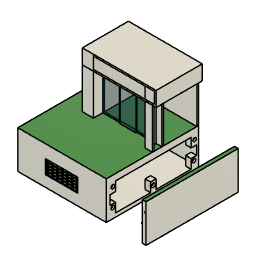
Test_Coffret_Conception Maison Energetique_1 v6(2) (Autodesk Fusion 360 design; units mm, degrees)
Autodesk Fusion 360 part; units mm, degrees
note: some values were not read from the file. Chosen so that the rebuilt part matches the saved one: which bodies a step acts on. Set by a fixed rule: which sketch regions a step uses.
(part 1 of 3)
sketch "Esquisse1" plane through (0, 0, 0) normal (0, 1, 0) x (1, 0, 0)
  line L0 (0, 0) -> (500, 0)
  line L1 (500, 0) -> (500, 500)
  line L2 (500, 500) -> (0, 500)
  line L3 (0, 500) -> (0, 0)
  dimension "d1" = 500
  dimension "d2" = 500
  constraint horizontal L0
  constraint vertical L1
  constraint horizontal L2
  constraint vertical L3
  constraint coincident L0.start L3.end
  measures "d1" distance of L0.start L0.end
  measures "d2" distance of L0.start L2.end
extrude "Extrusion1" add sketch "Esquisse1" along normal blind 40 makes body 1
sketch "Esquisse2" plane through (0, 40, 0) normal (0, 1, 0) x (-1, 0, 0)
  line L0 (0, -500) -> (0, 0)
  line L1 (0, 0) -> (-500, 0)
  line L2 (-500, 0) -> (-500, -500)
  line L3 (-500, -500) -> (0, -500)
  line L4 (-75, -500) -> (-500, -500)
  line L5 (-500, -500) -> (-500, -250)
  line L6 (-500, -250) -> (-75, -250)
  line L7 (-75, -250) -> (-75, -500)
  line L8 (-480, -480) -> (-480, -270)
  line L9 (-480, -270) -> (-95, -270)
  line L10 (-95, -270) -> (-95, -480)
  line L11 (-95, -480) -> (-480, -480)
  dimension "d5" = 20
  constraint horizontal L4
  constraint vertical L5
  constraint horizontal L6
  constraint vertical L7
  constraint midpoint L2 L5.end
  constraint coincident L3 L4.start
extrude "Extrusion2" add sketch "Esquisse2" along normal blind 400 contours L2 L3 L4 L5 L6 L7 bodies 1
sketch "Esquisse3" plane through (0, 440, 0) normal (0, 1, 0) x (-1, 0, 0)
  line L0 (-95, -270) -> (-95, -480)
  line L1 (-95, -480) -> (-480, -480)
  line L2 (-480, -480) -> (-480, -270)
  line L3 (-480, -270) -> (-95, -270)
  line L4 (-75, -250) -> (-500, -250)
  line L5 (-500, -250) -> (-500, -500)
  line L6 (-500, -500) -> (-75, -500)
  line L7 (-75, -500) -> (-75, -250)
  line L8 (-75, -500) -> (-500, -500)
  line L9 (-500, -500) -> (-500, -200)
  line L10 (-500, -200) -> (-75, -200)
  line L11 (-75, -200) -> (-75, -500)
  constraint horizontal L8
  constraint vertical L9
  constraint horizontal L10
  constraint vertical L11
  constraint coincident L6.end L7.start
extrude "Extrusion3" add sketch "Esquisse3" against normal blind 20 separate body contours L0 L1 L2 L3 | L4 L5 L6 L7 L8 L9 L11 | L4 L9 L10 L11 makes body 2
copy_body "Copier/Coller des corps1" bodies 2 makes body 3
move_body "Déplacer1" bodies 3 to x (1, 0, 0) y (0, 1, 0) z (0, 0, 1) at (0, -100, 0)
sketch "Esquisse4" plane through (0, 0, -250) normal (0, 0, 1) x (1, 0, 0)
  line L0 (75, 40) -> (500, 40)
  line L1 (500, 40) -> (500, 440)
  line L2 (500, 440) -> (75, 440)
  line L3 (75, 440) -> (75, 40)
  line L4 (75, 420) -> (500, 420)
  line L5 (500, 420) -> (500, 340)
  line L6 (500, 340) -> (75, 340)
  line L7 (75, 340) -> (75, 420)
  constraint horizontal L4
  constraint vertical L5
  constraint horizontal L6
  constraint vertical L7
  constraint coincident L1 L5.end
  constraint coincident L3 L4.start
extrude "Extrusion4" add sketch "Esquisse4" along normal blind 50 contours L1 L3 L4 L5 L6 L7 bodies 1 2 3
sketch "Esquisse5" plane through (0, 0, -200) normal (0, 0, 1) x (1, 0, 0)
  line L0 (500, 440) -> (75, 440)
  line L1 (75, 440) -> (75, 420)
  line L2 (75, 420) -> (75, 320)
  line L3 (75, 320) -> (500, 320)
  line L4 (500, 320) -> (500, 420)
  line L5 (500, 420) -> (500, 440)
  line L6 (95, 420) -> (95, 340)
  line L7 (95, 340) -> (480, 340)
  line L8 (480, 340) -> (480, 420)
  line L9 (480, 420) -> (95, 420)
  dimension "d12" = -20
extrude "Extrusion5" cut sketch "Esquisse5" against normal blind 280 contours L6 L7 L8 L9 bodies 1
ref_plane "Plan de construction1" through (287.5, 320, -225) normal (0, -1, 0) x (0, 0, -1)
split "Scinder1" by plane through (287.5, 320, -225) normal (0, -1, 0) bodies 1 makes body 4 at (166.6667, 0, -333.3333)
sketch "Esquisse6" plane through (0, 0, -200) normal (0, 0, 1) x (1, 0, 0)
  line L0 (95, 340) -> (95, 420)
  line L1 (95, 420) -> (480, 420)
  line L2 (480, 420) -> (480, 340)
  line L3 (480, 340) -> (95, 340)
  line L4 (500, 440) -> (75, 440)
  line L5 (75, 440) -> (75, 420)
  line L6 (75, 420) -> (75, 320)
  line L7 (75, 320) -> (500, 320)
  line L8 (500, 320) -> (500, 420)
  line L9 (500, 420) -> (500, 440)
  line L10 (95, 420) -> (480, 420)
  line L11 (480, 420) -> (480, 340)
  line L12 (480, 340) -> (95, 340)
  line L13 (95, 340) -> (95, 420)
  constraint horizontal L10
  constraint vertical L11
  constraint horizontal L12
  constraint vertical L13
  constraint coincident L2.end L3.start
  constraint coincident L0.end L1.start
extrude "Extrusion6" add sketch "Esquisse6" against normal blind 20 separate body contours L0 L1 L2 L3 L10 L11 L12 L13 makes body 5
ref_plane "Plan de construction2" through (250, 40, -250) normal (0, 1, 0) x (0, 0, 1)
split "Scinder2" by plane through (250, 40, -250) normal (0, 1, 0) bodies 4 makes body 6 at (358.3333, 133.3333, -500)
sketch "Esquisse7" plane through (0, 0, -250) normal (0, 0, 1) x (1, 0, 0)
  line L0 (500, 320) -> (75, 320)
  line L1 (75, 320) -> (75, 40)
  line L2 (75, 40) -> (500, 40)
  line L3 (500, 40) -> (500, 320)
  line L4 (188.1968, 40) -> (363.1968, 40)
  line L5 (363.1968, 40) -> (363.1968, 250)
  line L6 (363.1968, 250) -> (188.1968, 250)
  line L7 (188.1968, 250) -> (188.1968, 40)
  dimension "d19" = 175
  dimension "d20" = 210
  constraint horizontal L4
  constraint vertical L5
  constraint horizontal L6
  constraint vertical L7
  constraint coincident L2 L4.start
  measures "d19" distance of L4.start L4.end
  measures "d20" distance of L4.start L6.end
extrude "Extrusion7" cut sketch "Esquisse7" against normal blind 15 contours L2 L4 L5 L6 L7 bodies 6
sketch "Esquisse8" plane through (0, 0, -265) normal (0, 0, 1) x (1, 0, 0)
  line L0 (188.1968, 250) -> (188.1968, 40)
  line L1 (188.1968, 40) -> (363.1968, 40)
  line L2 (363.1968, 40) -> (363.1968, 250)
  line L3 (363.1968, 250) -> (188.1968, 250)
extrude "Extrusion8" add sketch "Esquisse8" along normal blind 20 bodies 6
sketch "Esquisse9" plane through (0, 40, 0) normal (0, 1, 0) x (-1, 0, 0)
  line L0 (-500, -500) -> (0, -500)
  line L1 (0, -500) -> (0, 0)
  line L2 (0, 0) -> (-500, 0)
  line L3 (-500, 0) -> (-500, -500)
  line L4 (-480, -270) -> (-450, -270)
  line L5 (-450, -270) -> (-450, -300)
  line L6 (-450, -300) -> (-480, -300)
  line L7 (-480, -300) -> (-480, -270)
  line L8 (-500, -320) -> (-500, -250)
  line L9 (-500, -250) -> (-430, -250)
  line L10 (-430, -250) -> (-430, -320)
  line L11 (-430, -320) -> (-500, -320)
  dimension "d25" = 30
  dimension "d26" = 30
  dimension "d27" = -20
  constraint horizontal L4
  constraint vertical L5
  constraint horizontal L6
  constraint vertical L7
  measures "d25" distance of L4.start L4.end
  measures "d26" distance of L4.start L6.end
extrude "Extrusion9" add sketch "Esquisse9" along normal blind 280 separate body contours L3 L8 L9 L10 L11 makes body 7
sketch "Esquisse10" plane through (0, 0, 0) normal (0, -1, 0) x (1, 0, 0)
  line L0 (0, 0) -> (0, -500)
  line L1 (0, -500) -> (500, -500)
  line L2 (500, -500) -> (500, 0)
  line L3 (500, 0) -> (0, 0)
  line L4 (480, -480) -> (480, -20)
  line L5 (480, -20) -> (20, -20)
  line L6 (20, -20) -> (20, -480)
  line L7 (20, -480) -> (480, -480)
  dimension "d30" = -20
extrude "Extrusion10" add sketch "Esquisse10" along normal blind 100 separate body makes body 8
sketch "Esquisse11" plane through (0, -100, 0) normal (0, -1, 0) x (1, 0, 0)
  line L0 (480, -480) -> (20, -480)
  line L1 (20, -480) -> (20, -20)
  line L2 (20, -20) -> (480, -20)
  line L3 (480, -20) -> (480, -480)
  line L4 (500, 0) -> (0, 0)
  line L5 (0, 0) -> (0, -500)
  line L6 (0, -500) -> (500, -500)
  line L7 (500, -500) -> (500, 0)
  line L8 (0, 0) -> (500, 0)
  line L9 (500, 0) -> (500, -500)
  line L10 (500, -500) -> (0, -500)
  line L11 (0, -500) -> (0, 0)
  constraint horizontal L8
  constraint vertical L9
  constraint horizontal L10
  constraint vertical L11
  constraint coincident L6.end L7.start
  constraint coincident L4.end L5.start
extrude "Extrusion11" add sketch "Esquisse11" along normal blind 20 separate body contours L0 L1 L2 L3 | L4 L5 L6 L7 L8 L9 L10 L11 makes body 9
sketch "Esquisse12" plane through (0, 0, 0) normal (0, -1, 0) x (1, 0, 0)
  line L0 (0, 0) -> (0, -500)
  line L1 (0, -500) -> (500, -500)
  line L2 (500, -500) -> (500, 0)
  line L3 (500, 0) -> (0, 0)
  line L4 (20, -171) -> (480.0003, -171)
  line L5 (480.0003, -171) -> (480.0003, -151)
  line L6 (480.0003, -151) -> (20, -151)
  line L7 (20, -151) -> (20, -171)
  dimension "d35" = 20
  constraint horizontal L4
  constraint vertical L5
  constraint horizontal L6
  constraint vertical L7
  measures "d35" distance of L4.start L6.end
extrude "Extrusion12" add sketch "Esquisse12" along normal blind 100 separate body contours L4 L5 L6 L7 makes body 10
move_body "Déplacer2" bodies 10 to x (1, 0, 0) y (0, 1, 0) z (0, 0, 1) at (0, 0, -50)
sketch "Esquisse13" plane through (0, 0, 0) normal (0, 0, 1) x (1, 0, 0)
  line L0 (500, 0) -> (0, 0)
  line L1 (0, 0) -> (0, -100)
  line L2 (0, -100) -> (500, -100)
  line L3 (500, -100) -> (500, 0)
  line L4 (480, -80) -> (480, -20)
  line L5 (480, -20) -> (20, -20)
  line L6 (20, -20) -> (20, -80)
  line L7 (20, -80) -> (480, -80)
  dimension "d38" = -20
extrude "Extrusion13" cut sketch "Esquisse13" against normal blind 20 contours L4 L5 L6 L7 bodies 8
sketch "Esquisse14" plane through (0, 0, -201) normal (0, 0, 1) x (1, 0, 0)
  line L0 (480.0003, 0) -> (20, 0)
  line L1 (20, 0) -> (20, -100)
  line L2 (20, -100) -> (480.0003, -100)
  line L3 (480.0003, -100) -> (480.0003, 0)
  line L4 (0, -50) -> (500, -50)
  line L5 (250, -50) -> (200, -50)
  line L6 (250, -50) -> (300, -50)
  line L7 (200, -50) -> (200, -25)
  line L8 (200, -50) -> (200, -75)
  line L9 (200, -25) -> (300, -25)
  line L10 (300, -25) -> (300, -75)
  line L11 (300, -75) -> (200, -75)
  line L12 (200, -75) -> (200, -25)
  dimension "d41" = 50
  dimension "d42" = 50
  dimension "d43" = 25
  dimension "d45" = 25
  constraint perpendicular L3 L4
  constraint midpoint L4 L5.start
  constraint parallel L4 L5
  constraint parallel L4 L6
  constraint perpendicular L0 L7
  constraint perpendicular L4 L8
  constraint horizontal L9
  constraint vertical L10
  constraint horizontal L11
  constraint vertical L12
  measures "d41" distance of L5.start L5.end
  measures "d42" distance of L5.start L6.end
  measures "d43" distance of L5.end L7.end
  measures "d45" distance of L5.end L8.end
extrude "Extrusion14" cut sketch "Esquisse14" against normal blind 20 contours L4 L5 L6 L8 L10 L11 L12 | L4 L5 L6 L7 L9 L10 L12 bodies 10
sketch "Esquisse15" plane through (0, 0, -480) normal (0, 0, 1) x (1, 0, 0)
  line L0 (480, 0) -> (20, 0)
  line L1 (20, 0) -> (20, -100)
  line L2 (20, -100) -> (480, -100)
  line L3 (480, -100) -> (480, 0)
  line L4 (230, -30) -> (270, -30)
  line L5 (270, -30) -> (270, -70)
  line L6 (270, -70) -> (230, -70)
  line L7 (230, -70) -> (230, -30)
  spline S0 degree 5 poles (250, -50) (249.4889, -49.5996) (248.5057, -48.7988) (247.1484, -47.5977) (245.5774, -45.9965) (244.0392, -43.9954) (242.9669, -41.9947) (242.4027, -39.9944) (242.3763, -37.9947) (242.8764, -35.9953) (243.8673, -33.9965) (245.0225, -32.3977) (246.0802, -31.1988) (246.8689, -30.3996) (247.2842, -30) knots 0 0 0 0 0 0 0.1 0.2 0.3 0.4 0.5 0.6 0.7 0.8 0.9 1 1 1 1 1 1
  spline S1 degree 5 poles (247.2842, -30) (247.159, -30.2933) (246.9356, -30.9388) (246.6822, -32.0838) (246.5187, -33.9882) (246.7472, -37.3065) (247.4945, -41.1841) (248.532, -45.1258) (249.4696, -48.2864) (250, -50) knots 0 0 0 0 0 0 0.2 0.4 0.6 0.8 1 1 1 1 1 1
  line L8 (248.6567, -45.6598) -> (251.3433, -54.3402)
  spline S2 degree 5 poles (249.6809, -50.207) (249.7158, -49.5586) (249.8078, -48.294) (250.0132, -46.4932) (250.4237, -44.2879) (251.1806, -41.88) (252.2045, -39.8541) (253.5194, -38.2446) (255.1423, -37.076) (257.0669, -36.3389) (259.2727, -36.0041) (261.2449, -36.0334) (262.8337, -36.2121) (263.9407, -36.3998) (264.5063, -36.5108) knots 0 0 0 0 0 0 0.1 0.2 0.3 0.4 0.5 0.6 0.7 0.8 0.9 1 1 1 1 1 1
  spline S3 degree 5 poles (264.5063, -36.5108) (264.1941, -36.5764) (263.5373, -36.7637) (262.454, -37.2128) (260.8003, -38.1712) (258.2131, -40.2617) (255.4654, -43.098) (252.8317, -46.2087) (250.7805, -48.7896) (249.6809, -50.207) knots 0 0 0 0 0 0 0.2 0.4 0.6 0.8 1 1 1 1 1 1
  line L9 (252.4658, -46.6172) -> (246.8961, -53.7967)
  spline S4 degree 5 poles (250, -50) (249.4889, -49.5996) (248.5057, -48.7988) (247.1484, -47.5977) (245.5774, -45.9965) (244.0392, -43.9954) (242.9669, -41.9947) (242.4027, -39.9944) (242.3763, -37.9947) (242.8764, -35.9953) (243.8673, -33.9965) (245.0225, -32.3977) (246.0802, -31.1988) (246.8689, -30.3996) (247.2842, -30) knots 0 0 0 0 0 0 0.1 0.2 0.3 0.4 0.5 0.6 0.7 0.8 0.9 1 1 1 1 1 1
  spline S5 degree 5 poles (247.2842, -30) (247.159, -30.2933) (246.9356, -30.9388) (246.6822, -32.0838) (246.5187, -33.9882) (246.7472, -37.3065) (247.4945, -41.1841) (248.532, -45.1258) (249.4696, -48.2864) (250, -50) knots 0 0 0 0 0 0 0.2 0.4 0.6 0.8 1 1 1 1 1 1
  line L10 (248.6567, -45.6598) -> (251.3433, -54.3402)
  spline S6 degree 5 poles (264.5063, -36.5108) (264.1941, -36.5764) (263.5373, -36.7637) (262.454, -37.2128) (260.8003, -38.1712) (258.2131, -40.2617) (255.4654, -43.098) (252.8317, -46.2087) (250.7805, -48.7896) (249.6809, -50.207) knots 0 0 0 0 0 0 0.2 0.4 0.6 0.8 1 1 1 1 1 1
  line L11 (252.4658, -46.6172) -> (246.8961, -53.7967)
  spline S7 degree 5 poles (249.6809, -50.207) (249.7158, -49.5586) (249.8078, -48.294) (250.0132, -46.4932) (250.4237, -44.2879) (251.1806, -41.88) (252.2045, -39.8541) (253.5194, -38.2446) (255.1423, -37.076) (257.0669, -36.3389) (259.2727, -36.0041) (261.2449, -36.0334) (262.8337, -36.2121) (263.9407, -36.3998) (264.5063, -36.5108) knots 0 0 0 0 0 0 0.1 0.2 0.3 0.4 0.5 0.6 0.7 0.8 0.9 1 1 1 1 1 1
  spline S8 degree 5 poles (250.0313, -49.9578) (250.4317, -49.4466) (251.2325, -48.4635) (252.4336, -47.1062) (254.0348, -45.5352) (256.0359, -43.9969) (258.0366, -42.9247) (260.0369, -42.3604) (262.0367, -42.334) (264.036, -42.8342) (266.0349, -43.8251) (267.6336, -44.9803) (268.8326, -46.038) (269.6318, -46.8267) (270.0313, -47.242) knots 0 0 0 0 0 0 0.1 0.2 0.3 0.4 0.5 0.6 0.7 0.8 0.9 1 1 1 1 1 1
  spline S9 degree 5 poles (270.0313, -47.242) (269.738, -47.1167) (269.0925, -46.8934) (267.9476, -46.64) (266.0432, -46.4765) (262.7249, -46.705) (258.8472, -47.4523) (254.9056, -48.4898) (251.745, -49.4274) (250.0313, -49.9578) knots 0 0 0 0 0 0 0.2 0.4 0.6 0.8 1 1 1 1 1 1
  line L12 (254.3715, -48.6145) -> (245.6911, -51.301)
  spline S10 degree 5 poles (263.5206, -64.464) (263.4549, -64.1519) (263.2676, -63.4951) (262.8185, -62.4118) (261.8601, -60.758) (259.7696, -58.1709) (256.9334, -55.4232) (253.8226, -52.7894) (251.2417, -50.7382) (249.8244, -49.6387) knots 0 0 0 0 0 0 0.2 0.4 0.6 0.8 1 1 1 1 1 1
  line L13 (253.4142, -52.4235) -> (246.2346, -46.8539)
  spline S11 degree 5 poles (249.8244, -49.6387) (250.4727, -49.6735) (251.7374, -49.7656) (253.5381, -49.9709) (255.7434, -50.3815) (258.1513, -51.1384) (260.1772, -52.1622) (261.7867, -53.4771) (262.9554, -55.1001) (263.6925, -57.0247) (264.0273, -59.2305) (263.998, -61.2027) (263.8192, -62.7915) (263.6315, -63.8985) (263.5206, -64.464) knots 0 0 0 0 0 0 0.1 0.2 0.3 0.4 0.5 0.6 0.7 0.8 0.9 1 1 1 1 1 1
  spline S12 degree 5 poles (250, -50) (249.4889, -49.5996) (248.5057, -48.7988) (247.1484, -47.5977) (245.5774, -45.9965) (244.0392, -43.9954) (242.9669, -41.9947) (242.4027, -39.9944) (242.3763, -37.9947) (242.8764, -35.9953) (243.8673, -33.9965) (245.0225, -32.3977) (246.0802, -31.1988) (246.8689, -30.3996) (247.2842, -30) knots 0 0 0 0 0 0 0.1 0.2 0.3 0.4 0.5 0.6 0.7 0.8 0.9 1 1 1 1 1 1
  spline S13 degree 5 poles (247.2842, -30) (247.159, -30.2933) (246.9356, -30.9388) (246.6822, -32.0838) (246.5187, -33.9882) (246.7472, -37.3065) (247.4945, -41.1841) (248.532, -45.1258) (249.4696, -48.2864) (250, -50) knots 0 0 0 0 0 0 0.2 0.4 0.6 0.8 1 1 1 1 1 1
  line L14 (248.6567, -45.6598) -> (251.3433, -54.3402)
  spline S14 degree 5 poles (249.6809, -50.207) (249.7158, -49.5586) (249.8078, -48.294) (250.0132, -46.4932) (250.4237, -44.2879) (251.1806, -41.88) (252.2045, -39.8541) (253.5194, -38.2446) (255.1423, -37.076) (257.0669, -36.3389) (259.2727, -36.0041) (261.2449, -36.0334) (262.8337, -36.2121) (263.9407, -36.3998) (264.5063, -36.5108) knots 0 0 0 0 0 0 0.1 0.2 0.3 0.4 0.5 0.6 0.7 0.8 0.9 1 1 1 1 1 1
  spline S15 degree 5 poles (264.5063, -36.5108) (264.1941, -36.5764) (263.5373, -36.7637) (262.454, -37.2128) (260.8003, -38.1712) (258.2131, -40.2617) (255.4654, -43.098) (252.8317, -46.2087) (250.7805, -48.7896) (249.6809, -50.207) knots 0 0 0 0 0 0 0.2 0.4 0.6 0.8 1 1 1 1 1 1
  line L15 (252.4658, -46.6172) -> (246.8961, -53.7967)
  spline S16 degree 5 poles (250.0313, -49.9578) (250.4317, -49.4466) (251.2325, -48.4635) (252.4336, -47.1062) (254.0348, -45.5352) (256.0359, -43.9969) (258.0366, -42.9247) (260.0369, -42.3604) (262.0367, -42.334) (264.036, -42.8342) (266.0349, -43.8251) (267.6336, -44.9803) (268.8326, -46.038) (269.6318, -46.8267) (270.0313, -47.242) knots 0 0 0 0 0 0 0.1 0.2 0.3 0.4 0.5 0.6 0.7 0.8 0.9 1 1 1 1 1 1
  spline S17 degree 5 poles (270.0313, -47.242) (269.738, -47.1167) (269.0925, -46.8934) (267.9476, -46.64) (266.0432, -46.4765) (262.7249, -46.705) (258.8472, -47.4523) (254.9056, -48.4898) (251.745, -49.4274) (250.0313, -49.9578) knots 0 0 0 0 0 0 0.2 0.4 0.6 0.8 1 1 1 1 1 1
  line L16 (254.3715, -48.6145) -> (245.6911, -51.301)
  spline S18 degree 5 poles (249.8244, -49.6387) (250.4727, -49.6735) (251.7374, -49.7656) (253.5381, -49.9709) (255.7434, -50.3815) (258.1513, -51.1384) (260.1772, -52.1622) (261.7867, -53.4771) (262.9554, -55.1001) (263.6925, -57.0247) (264.0273, -59.2305) (263.998, -61.2027) (263.8192, -62.7915) (263.6315, -63.8985) (263.5206, -64.464) knots 0 0 0 0 0 0 0.1 0.2 0.3 0.4 0.5 0.6 0.7 0.8 0.9 1 1 1 1 1 1
  spline S19 degree 5 poles (263.5206, -64.464) (263.4549, -64.1519) (263.2676, -63.4951) (262.8185, -62.4118) (261.8601, -60.758) (259.7696, -58.1709) (256.9334, -55.4232) (253.8226, -52.7894) (251.2417, -50.7382) (249.8244, -49.6387) knots 0 0 0 0 0 0 0.2 0.4 0.6 0.8 1 1 1 1 1 1
  line L17 (253.4142, -52.4235) -> (246.2346, -46.8539)
  spline S20 degree 5 poles (249.8118, -49.3682) (250.3847, -49.6738) (251.4919, -50.2917) (253.0372, -51.2388) (254.8624, -52.5429) (256.7248, -54.2465) (258.1282, -56.0306) (259.0312, -57.9025) (259.4044, -59.8673) (259.2591, -61.9231) (258.6303, -64.0637) (257.7703, -65.8388) (256.9369, -67.2031) (256.2989, -68.1272) (255.9593, -68.5928) knots 0 0 0 0 0 0 0.1 0.2 0.3 0.4 0.5 0.6 0.7 0.8 0.9 1 1 1 1 1 1
  spline S21 degree 5 poles (255.9593, -68.5928) (256.0317, -68.2822) (256.1395, -67.6077) (256.1903, -66.4361) (256.0206, -64.5323) (255.2194, -61.3041) (253.8101, -57.6151) (252.1039, -53.9135) (250.6317, -50.9637) (249.8118, -49.3682) knots 0 0 0 0 0 0 0.2 0.4 0.6 0.8 1 1 1 1 1 1
  line L18 (251.8883, -53.4092) -> (247.7353, -45.3272)
  spline S22 degree 5 poles (250.0901, -49.109) (250.1684, -49.7536) (250.2973, -51.015) (250.4078, -52.824) (250.3865, -55.0671) (250.0592, -57.5699) (249.4026, -59.7428) (248.3872, -61.5561) (246.9918, -62.9889) (245.2245, -64.049) (243.1104, -64.7617) (241.163, -65.0753) (239.5673, -65.1752) (238.4445, -65.1826) (237.8683, -65.1715) knots 0 0 0 0 0 0 0.1 0.2 0.3 0.4 0.5 0.6 0.7 0.8 0.9 1 1 1 1 1 1
  spline S23 degree 5 poles (237.8683, -65.1715) (238.1643, -65.0527) (238.7786, -64.7541) (239.7674, -64.1237) (241.2297, -62.8927) (243.4145, -60.3848) (245.6279, -57.1144) (247.6815, -53.5936) (249.2534, -50.6957) (250.0901, -49.109) knots 0 0 0 0 0 0 0.2 0.4 0.6 0.8 1 1 1 1 1 1
  line L19 (247.9709, -53.1278) -> (252.2093, -45.0902)
  spline S24 degree 5 poles (249.7883, -49.4152) (249.4827, -49.9881) (248.8648, -51.0954) (247.9177, -52.6406) (246.6136, -54.4658) (244.91, -56.3282) (243.1259, -57.7316) (241.254, -58.6346) (239.2892, -59.0079) (237.2334, -58.8625) (235.0928, -58.2338) (233.3177, -57.3737) (231.9534, -56.5403) (231.0293, -55.9023) (230.5637, -55.5627) knots 0 0 0 0 0 0 0.1 0.2 0.3 0.4 0.5 0.6 0.7 0.8 0.9 1 1 1 1 1 1
  spline S25 degree 5 poles (230.5637, -55.5627) (230.8743, -55.6352) (231.5488, -55.743) (232.7204, -55.7938) (234.6242, -55.6241) (237.8524, -54.8228) (241.5414, -53.4135) (245.243, -51.7073) (248.1928, -50.2351) (249.7883, -49.4152) knots 0 0 0 0 0 0 0.2 0.4 0.6 0.8 1 1 1 1 1 1
  line L20 (245.7473, -51.4918) -> (253.8293, -47.3387)
  spline S26 degree 5 poles (250.0475, -49.6935) (249.4029, -49.7718) (248.1415, -49.9008) (246.3325, -50.0112) (244.0894, -49.9899) (241.5866, -49.6626) (239.4137, -49.0061) (237.6004, -47.9907) (236.1676, -46.5953) (235.1075, -44.8279) (234.3948, -42.7138) (234.0812, -40.7664) (233.9813, -39.1708) (233.9739, -38.0479) (233.985, -37.4718) knots 0 0 0 0 0 0 0.1 0.2 0.3 0.4 0.5 0.6 0.7 0.8 0.9 1 1 1 1 1 1
  spline S27 degree 5 poles (233.985, -37.4718) (234.1038, -37.7677) (234.4024, -38.3821) (235.0328, -39.3709) (236.2638, -40.8331) (238.7717, -43.0179) (242.0421, -45.2314) (245.5629, -47.2849) (248.4608, -48.8568) (250.0475, -49.6935) knots 0 0 0 0 0 0 0.2 0.4 0.6 0.8 1 1 1 1 1 1
  line L21 (246.0287, -47.5744) -> (254.0663, -51.8127)
  line L22 (272, -28) -> (272, -72)
  line L23 (272, -72) -> (228, -72)
  line L24 (228, -72) -> (228, -28)
  line L25 (228, -28) -> (272, -28)
  point P0 (242.4871, -39.58)
  point P1 (253.9073, -38.0761)
  point P2 (242.4871, -39.58)
  point P3 (253.9073, -38.0761)
  point P4 (260.4513, -42.4449)
  point P5 (261.9552, -53.8651)
  point P6 (242.4871, -39.58)
  point P7 (261.9552, -53.8651)
  point P8 (260.4513, -42.4449)
  point P9 (253.9073, -38.0761)
  point P10 (259.0199, -58.3253)
  point P11 (237.3671, -47.6379)
  point P12 (240.8312, -58.6234)
  point P13 (248.0344, -61.7894)
  dimension "d50" = -2
  constraint horizontal L4
  constraint vertical L5
  constraint horizontal L6
  constraint vertical L7
  constraint coincident L4 S0.end
  constraint midpoint S0.start L8
  constraint midpoint S2.start L9
  constraint midpoint S0.start L10
  constraint midpoint S2.start L11
  constraint midpoint S8.start L12
  constraint midpoint S10.end L13
  constraint midpoint S0.start L14
  constraint midpoint S2.start L15
  constraint midpoint S8.start L16
  constraint midpoint S10.end L17
  constraint midpoint S20.start L18
  constraint midpoint S22.start L19
  constraint midpoint S24.start L20
  constraint midpoint S26.start L21
extrude "Extrusion15" cut sketch "Esquisse15" against normal blind 20 contours S0 S1 S2 S4 S5 S7 L13 S12 S13 S14 L17 S25 L20 S27 L21 | S0 S4 L13 S12 L17 S27 | S1 L8 S2 S3 S5 L10 S6 S7 S13 L14 S14 S15 S20 L18 S22 S23 L19 L20 | L5 S8 S9 S11 S16 S17 S18 S20 | S0 S4 S12 S25 L20 S26 S27 | S1 L8 S5 L10 S13 L14 S21 L18 L20 | S1 L8 S5 L10 S13 L14 S21 L18 S23 L19 L20 | S3 L9 S6 L11 S15 L15 L20 | S9 L12 S10 S11 S17 L16 S18 S19 S20 | L12 L16 S25 L20 | L12 L16 S24 L20 S26 | S20 S23 L19 L20 | L9 L11 L15 S20 S22 L20 | L12 L16 S24 S25 | S10 S19 S20 S21 S22 | L12 L16 S23 L19 | L9 L11 L12 L15 L16 S23 L19 | S1 L8 S5 L10 S9 L12 S13 L14 S17 L16 S21 L18 S22 | S2 S7 L12 S14 L16 L19 | S0 L8 S3 L9 S4 L10 S6 L11 L12 S12 L14 S15 L15 L16 S22 S23 | S2 L9 L11 S7 L12 S14 L15 L16 L19 | S1 L8 S3 L9 S5 L10 S6 L11 S8 L12 S10 L13 S13 L14 S15 L15 S16 L16 S19 L17 S21 L18 | S0 S3 L9 S4 S6 L11 L12 S12 S15 L15 L16 bodies 8
extrude "Extrusion16" add sketch "Esquisse15" along normal blind 2 and the other way blind 22 separate body contours L22 L23 L24 L25 makes body 11
sketch "Esquisse16" plane through (0, 0, 0) normal (0, 1, 0) x (1, 0, 0)
  line L0 (0, -500) -> (500, -500)
  line L1 (500, -500) -> (500, -1000)
  line L2 (500, -1000) -> (0, -1000)
  line L3 (0, -1000) -> (0, -500)
  dimension "d55" = 500
  dimension "d56" = 500
  constraint horizontal L0
  constraint vertical L1
  constraint horizontal L2
  constraint vertical L3
  measures "d55" distance of L0.start L0.end
  measures "d56" distance of L0.start L2.end
extrude "Extrusion17" add sketch "Esquisse16" along normal blind 20 separate body makes body 12
sketch "Esquisse17" plane through (0, 20, 0) normal (0, 1, 0) x (-1, 0, 0)
  line L0 (0, 1000) -> (-500, 1000)
  line L1 (-500, 1000) -> (-500, 500)
  line L2 (-500, 500) -> (0, 500)
  line L3 (0, 500) -> (0, 1000)
  line L4 (-500, 500) -> (-100, 500)
  line L5 (-100, 500) -> (-100, 750)
  line L6 (-100, 750) -> (-500, 750)
  line L7 (-500, 750) -> (-500, 500)
  line L8 (-491, 741) -> (-491, 509)
  line L9 (-491, 509) -> (-109, 509)
  line L10 (-109, 509) -> (-109, 741)
  line L11 (-109, 741) -> (-491, 741)
  dimension "d59" = 400
  dimension "d60" = 250
  dimension "d61" = -9
  constraint horizontal L4
  constraint vertical L5
  constraint horizontal L6
  constraint vertical L7
  constraint coincident L1.end L2.start
  measures "d59" distance of L1.end L4.end
  measures "d60" distance of L1.end L6.end
extrude "Extrusion18" add sketch "Esquisse17" along normal blind 300 contours L1 L2 L4 L5 L6 L7 bodies 12
sketch "Esquisse18" plane through (0, 20, 0) normal (0, 1, 0) x (-1, 0, 0)
  line L0 (-491, 741) -> (-491, 509)
  line L1 (-491, 509) -> (-109, 509)
  line L2 (-109, 509) -> (-109, 741)
  line L3 (-109, 741) -> (-491, 741)
  line L4 (-100, 750) -> (-160, 750)
  line L5 (-160, 750) -> (-160, 690)
  line L6 (-160, 690) -> (-100, 690)
  line L7 (-100, 690) -> (-100, 750)
  line L8 (-109, 741) -> (-151, 741)
  line L9 (-151, 741) -> (-151, 699)
  line L10 (-151, 699) -> (-109, 699)
  line L11 (-109, 699) -> (-109, 741)
  dimension "d64" = 60
  dimension "d65" = 60
  dimension "d66" = -9
  constraint horizontal L4
  constraint vertical L5
  constraint horizontal L6
  constraint vertical L7
  measures "d64" distance of L4.start L4.end
  measures "d65" distance of L4.start L6.end
extrude "Extrusion19" add sketch "Esquisse18" along normal blind 300 contours L2 L3 L5 L6 L9 L10 bodies 12
sketch "Esquisse19" plane through (0, 20, 0) normal (0, 1, 0) x (-1, 0, 0)
  line L0 (-109, 690) -> (-160, 690)
  line L1 (-160, 690) -> (-160, 741)
  line L2 (-160, 741) -> (-491, 741)
  line L3 (-491, 741) -> (-491, 509)
  line L4 (-491, 509) -> (-109, 509)
  line L5 (-109, 509) -> (-109, 690)
  line L6 (-500, 750) -> (-440, 750)
  line L7 (-440, 750) -> (-440, 690)
  line L8 (-440, 690) -> (-500, 690)
  line L9 (-500, 690) -> (-500, 750)
  line L10 (-491, 699) -> (-491, 741)
  line L11 (-491, 741) -> (-449, 741)
  line L12 (-449, 741) -> (-449, 699)
  line L13 (-449, 699) -> (-491, 699)
  dimension "d69" = 60
  dimension "d70" = 60
  dimension "d71" = 9
  constraint horizontal L6
  constraint vertical L7
  constraint horizontal L8
  constraint vertical L9
  measures "d69" distance of L6.start L6.end
  measures "d70" distance of L6.start L8.end
extrude "Extrusion20" add sketch "Esquisse19" along normal blind 300 contours L2 L3 L7 L8 L12 L13 bodies 12
sketch "Esquisse20" plane through (0, 20, 0) normal (0, 1, 0) x (-1, 0, 0)
  line L0 (-440, 690) -> (-491, 690)
  line L1 (-491, 690) -> (-491, 509)
  line L2 (-491, 509) -> (-109, 509)
  line L3 (-109, 509) -> (-109, 690)
  line L4 (-109, 690) -> (-160, 690)
  line L5 (-160, 690) -> (-160, 741)
  line L6 (-160, 741) -> (-440, 741)
  line L7 (-440, 741) -> (-440, 690)
  line L8 (-160, 690) -> (-440, 690)
  line L9 (-160, 699) -> (-440, 699.0366)
  dimension "d74" = 280
  constraint coincident L4.end L5.start
  constraint coincident L0.start L7.end
  constraint coincident L5 L9.start
  measures "d74" distance of L9.start L9.end
extrude "Extrusion21" add sketch "Esquisse20" along normal blind 300 contours L5 L7 L8 L9 bodies 12
sketch "Esquisse21" plane through (0, 0, 750) normal (0, 0, 1) x (1, 0, 0)
  line L0 (100, 20) -> (500, 20)
  line L1 (500, 20) -> (500, 320)
  line L2 (500, 320) -> (100, 320)
  line L3 (100, 320) -> (100, 20)
  line L4 (160, 320) -> (440, 320)
  line L5 (440, 320) -> (440, 20)
  line L6 (440, 20) -> (160, 20)
  line L7 (160, 20) -> (160, 320)
  dimension "d77" = 280
  dimension "d78" = 300
  constraint horizontal L4
  constraint vertical L5
  constraint horizontal L6
  constraint vertical L7
  constraint coincident L2 L4.start
  measures "d77" distance of L4.start L4.end
  measures "d78" distance of L4.start L6.end
extrude "Extrusion22" cut sketch "Esquisse21" against normal blind 30 contours L0 L2 L4 L5 L6 L7 bodies 12
sketch "Esquisse22" plane through (0, 20, 0) normal (0, 1, 0) x (-1, 0, 0)
  line L0 (-109, 690) -> (-491, 690)
  line L1 (-491, 690) -> (-491, 509)
  line L2 (-491, 509) -> (-109, 509)
  line L3 (-109, 509) -> (-109, 690)
  line L4 (-100, 500) -> (-160, 500)
  line L5 (-160, 500) -> (-160, 560)
  line L6 (-160, 560) -> (-100, 560)
  line L7 (-100, 560) -> (-100, 500)
  line L8 (-109, 551) -> (-109, 509)
  line L9 (-109, 509) -> (-151, 509)
  line L10 (-151, 509) -> (-151, 551)
  line L11 (-151, 551) -> (-109, 551)
  dimension "d81" = 60
  dimension "d82" = 60
  dimension "d83" = 9
  constraint horizontal L4
  constraint vertical L5
  constraint horizontal L6
  constraint vertical L7
  measures "d81" distance of L4.start L4.end
  measures "d82" distance of L4.start L6.end
extrude "Extrusion23" add sketch "Esquisse22" along normal blind 300 contours L2 L3 L5 L6 L10 L11 bodies 12
sketch "Esquisse23" plane through (-0.0912, 0, 698.9791) normal (-0.00013, 0, 1) x (1, 0, 0.00013)
  line L0 (160.0912, 20) -> (440.0912, 20)
  line L1 (440.0912, 20) -> (440.0912, 320)
  line L2 (440.0912, 320) -> (160.0912, 320)
  line L3 (160.0912, 320) -> (160.0912, 20)
  line L4 (100, 320) -> (500, 320)
  line L5 (500, 320) -> (500, 240)
  line L6 (500, 240) -> (100, 240)
  line L7 (100, 240) -> (100, 320)
  line L8 (491, 249) -> (109, 249)
  line L9 (109, 249) -> (109, 311)
  line L10 (109, 311) -> (491, 311)
  line L11 (491, 311) -> (491, 249)
  dimension "d86" = 400
  dimension "d87" = 80
  dimension "d88" = 9
  constraint horizontal L4
  constraint vertical L5
  constraint horizontal L6
  constraint vertical L7
  measures "d86" distance of L4.start L4.end
  measures "d87" distance of L4.start L6.end
extrude "Extrusion24" add sketch "Esquisse23" along normal blind 51 and the other way blind 199 contours L3 L4 L6 L7 L8 L9 L10 | L1 L3 L6 L8 | L1 L4 L5 L6 L8 L10 L11 | L1 L2 L3 L4 L10 bodies 12
extrude "Extrusion25" cut 1 faces at (253.3333, 290.3333, 699.0122) along direction (0.00013, 0, -1) blind 40 on bodies 12 bodies 12
sketch "Esquisse24" plane through (0, 249, 0) normal (0, 1, 0) x (-1, 0, 0)
  line L0 (-160, 750) -> (-159.9169, 750)
  line L1 (-159.9169, 750) -> (-490.9021, 750.0432)
  line L2 (-490.9021, 750.0432) -> (-490.9021, 750)
  line L3 (-490.9021, 750) -> (-440, 750)
  line L4 (-440, 750) -> (-440, 699.0366)
  line L5 (-440, 699.0366) -> (-440.0012, 690)
  line L6 (-440.0012, 690) -> (-490.91, 690)
  line L7 (-490.91, 690) -> (-490.9336, 509)
  line L8 (-490.9336, 509) -> (-160, 509)
  line L9 (-160, 509) -> (-160, 560)
  line L10 (-160, 560) -> (-109, 560)
  line L11 (-109, 560) -> (-109, 690)
  line L12 (-109, 690) -> (-160.0012, 690)
  line L13 (-160.0012, 690) -> (-160, 699)
  line L14 (-160, 699) -> (-160, 750)
  line L15 (-160, 750) -> (-440, 750)
  line L16 (-440, 750) -> (-440, 741)
  line L17 (-440, 741) -> (-160, 741)
  line L18 (-160, 741) -> (-160, 750)
  dimension "d95" = 280
  dimension "d96" = 9
  constraint horizontal L15
  constraint vertical L16
  constraint horizontal L17
  constraint vertical L18
  constraint coincident L0.start L14.end
  measures "d95" distance of L0.start L3.end
  measures "d96" distance of L0.start L17.end
extrude "Extrusion26" add sketch "Esquisse24" along normal blind 62 separate body contours L4 L14 L15 L16 L17 L18 makes body 13
sketch "Esquisse25" plane through (-0.0912, 0, 698.9791) normal (-0.00013, 0, 1) x (1, 0, 0.00013)
  line L0 (440.0912, 240) -> (160.0912, 240)
  line L1 (160.0912, 240) -> (160.0912, 20)
  line L2 (160.0912, 20) -> (440.0912, 20)
  line L3 (440.0912, 20) -> (440.0912, 240)
  line L4 (160.0912, 190.8645) -> (440.0912, 190.8645) construction
  line L5 (300.0912, 190.8645) -> (300.0912, 240) construction
  line L6 (300.0912, 190.8645) -> (300.0912, 17.9885) construction
  line L7 (300.0912, 240) -> (345.0912, 240)
  line L8 (345.0912, 240) -> (345.0912, 20)
  line L9 (345.0912, 20) -> (300.0912, 20)
  line L10 (300.0912, 20) -> (300.0912, 240)
  line L11 (300.0912, 240) -> (255.0912, 240)
  line L12 (255.0912, 240) -> (255.0912, 20)
  line L13 (255.0912, 20) -> (300.0912, 20)
  line L14 (300.0912, 20) -> (300.0912, 240)
  dimension "d99" = 45
  dimension "d100" = 220
  dimension "d101" = 220
  constraint coincident L1 L4.start
  constraint coincident L3 L4.end
  constraint perpendicular L3 L4
  constraint midpoint L4 L5.start
  constraint midpoint L0 L5.end
  constraint perpendicular L2 L6
  constraint horizontal L7
  constraint vertical L8
  constraint horizontal L9
  constraint vertical L10
  constraint horizontal L11
  constraint vertical L12
  constraint horizontal L13
  constraint vertical L14
  measures "d99" distance of L5.end L7.end
  measures "d100" distance of L5.end L9.end
  measures "d101" distance of L5.end L9.end
extrude "Extrusion27" add sketch "Esquisse25" along normal blind 5 contours L0 L2 L7 L8 L9 L10 L14 | L0 L2 L10 L11 L12 L13 L14 bodies 12
sketch "Esquisse26" plane through (100, 0, 0) normal (-1, 0, 0) x (0, 0, 1)
  line L0 (749.9922, 320) -> (749.9922, 240)
  line L1 (749.9922, 240) -> (500, 240)
  line L2 (500, 240) -> (500, 20)
  line L3 (500, 20) -> (750, 20)
  line L4 (750, 20) -> (750, 320)
  line L5 (750, 320) -> (749.9922, 320)
  line L6 (500, 240) -> (560, 240) construction
  line L7 (560, 240) -> (690, 240)
  line L8 (690, 240) -> (690, 20)
  line L9 (690, 20) -> (560, 20)
  line L10 (560, 20) -> (560, 240)
  dimension "d104" = 60
  dimension "d105" = 130
  dimension "d106" = 220
  constraint coincident L1.end L2.start
  constraint perpendicular L2 L6
  constraint horizontal L7
  constraint vertical L8
  constraint horizontal L9
  constraint vertical L10
  measures "d104" distance of L1.end L6.end
  measures "d105" distance of L6.end L7.end
  measures "d106" distance of L6.end L9.end
extrude "Extrusion28" cut sketch "Esquisse26" against normal blind 70 contours L1 L3 L7 L8 L9 L10 bodies 12
sketch "Esquisse27" plane through (0, 20, 0) normal (0, 1, 0) x (-1, 0, 0)
  line L0 (-345, 699.0242) -> (-344.9993, 704.0242)
  line L1 (-344.9993, 704.0242) -> (-254.9993, 704.0124)
  line L2 (-254.9993, 704.0124) -> (-255, 699.0124)
  line L3 (-255, 699.0124) -> (-160, 699)
  line L4 (-160, 699) -> (-160, 750)
  line L5 (-160, 750) -> (-100, 750)
  line L6 (-100, 750) -> (-100, 690)
  line L7 (-100, 690) -> (-491, 690)
  line L8 (-491, 690) -> (-491, 509)
  line L9 (-491, 509) -> (-160, 509)
  line L10 (-160, 509) -> (-160, 560)
  line L11 (-160, 560) -> (-100, 560)
  line L12 (-100, 560) -> (-100, 500)
  line L13 (-100, 500) -> (0, 500)
  line L14 (0, 500) -> (0, 1000)
  line L15 (0, 1000) -> (-500, 1000)
  line L16 (-500, 1000) -> (-500, 750)
  line L17 (-500, 750) -> (-440, 750)
  line L18 (-440, 750) -> (-440, 699.0366)
  line L19 (-440, 699.0366) -> (-345, 699.0242)
  line L20 (-160, 560) -> (-151, 560)
  line L21 (-151, 560) -> (-151, 690)
  line L22 (-151, 690) -> (-160, 690)
  line L23 (-160, 690) -> (-160, 560)
  dimension "d109" = 9
  dimension "d110" = 130
  constraint horizontal L20
  constraint vertical L21
  constraint horizontal L22
  constraint vertical L23
  constraint coincident L10.end L11.start
  measures "d109" distance of L10.end L20.end
  measures "d110" distance of L10.end L22.end
extrude "Extrusion29" add sketch "Esquisse27" along normal blind 220 contours L7 L11 L20 L21 L22 L23 bodies 12
sketch "Esquisse28" plane through (151, 0, 0) normal (-1, 0, 0) x (0, 0, 1)
  line L0 (560, 20) -> (690, 20)
  line L1 (690, 20) -> (690, 240)
  line L2 (690, 240) -> (560, 240)
  line L3 (560, 240) -> (560, 20)
  line L4 (625, 240) -> (657.5, 240)
  line L5 (657.5, 240) -> (657.5, 20)
  line L6 (657.5, 20) -> (625, 20)
  line L7 (625, 20) -> (625, 240)
  line L8 (625, 240) -> (592.5, 240)
  line L9 (592.5, 240) -> (592.5, 20)
  line L10 (592.5, 20) -> (625, 20)
  line L11 (625, 20) -> (625, 240)
  dimension "d113" = 32.5
  dimension "d114" = 220
  dimension "d115" = 220
  constraint horizontal L4
  constraint vertical L5
  constraint horizontal L6
  constraint vertical L7
  constraint midpoint L2 L4.start
  constraint horizontal L8
  constraint vertical L9
  constraint horizontal L10
  constraint vertical L11
  measures "d113" distance of L4.start L4.end
  measures "d114" distance of L4.start L6.end
  measures "d115" distance of L4.start L6.end
extrude "Extrusion30" add sketch "Esquisse28" along normal blind 5 contours L0 L2 L7 L8 L9 L10 L11 | L0 L2 L4 L5 L6 L7 L11 bodies 12
split "Scinder3" by plane through (160, 240, 699) normal (0, -1, 0) bodies 12 makes body 14 at (166.6667, 0, 666.6667)
sketch "Esquisse29" plane through (500, 0, 0) normal (1, 0, 0) x (0, 0, -1)
  line L0 (-500, 240) -> (-750, 240)
  line L1 (-750, 240) -> (-750, 20)
  line L2 (-750, 20) -> (-1000, 20)
  line L3 (-1000, 20) -> (-1000, 0)
  line L4 (-1000, 0) -> (-500, 0)
  line L5 (-500, 0) -> (-500, 240)
  line L6 (-1000, 0) -> (-500, 0)
  line L7 (-500, 0) -> (-500, -15)
  line L8 (-500, -15) -> (-1000, -15)
  line L9 (-1000, -15) -> (-1000, 0)
  dimension "d118" = 500
  dimension "d119" = 15
  constraint horizontal L6
  constraint vertical L7
  constraint horizontal L8
  constraint vertical L9
  constraint coincident L3.end L4.start
  measures "d118" distance of L3.end L4.end
  measures "d119" distance of L3.end L8.end
extrude "Extrusion31" add sketch "Esquisse29" against normal blind 500 contours L4 L6 L7 L8 L9 bodies 14
sketch "Esquisse30" plane through (500, 0, 0) normal (1, 0, 0) x (0, 0, -1)
  line L0 (-500, 240) -> (-750, 240)
  line L1 (-750, 240) -> (-750, 20)
  line L2 (-750, 20) -> (-1000, 20)
  line L3 (-1000, 20) -> (-1000, -15)
  line L4 (-1000, -15) -> (-500, -15)
  line L5 (-500, -15) -> (-500, 240)
  line L6 (-1000, -15) -> (-500, -15)
  line L7 (-500, -15) -> (-500, -185)
  line L8 (-500, -185) -> (-1000, -185)
  line L9 (-1000, -185) -> (-1000, -15)
  line L10 (-980, -165) -> (-980, -35)
  line L11 (-980, -35) -> (-520, -35)
  line L12 (-520, -35) -> (-520, -165)
  line L13 (-520, -165) -> (-980, -165)
  dimension "d122" = 500
  dimension "d123" = 170
  dimension "d124" = 20
  constraint horizontal L6
  constraint vertical L7
  constraint horizontal L8
  constraint vertical L9
  constraint coincident L3.end L4.start
  measures "d122" distance of L3.end L4.end
  measures "d123" distance of L3.end L8.end
extrude "Extrusion32" add sketch "Esquisse30" against normal blind 500 contours L4 L6 L7 L8 L9 bodies 14
sketch "Esquisse31" plane through (0, 0, 1000) normal (0, 0, 1) x (1, 0, 0)
  line L0 (500, -185) -> (500, 20)
  line L1 (500, 20) -> (0, 20)
  line L2 (0, 20) -> (0, -185)
  line L3 (0, -185) -> (500, -185)
  line L4 (0, 20) -> (0, -15) construction
  line L5 (0, -15) -> (500, -15)
  line L6 (500, -15) -> (500, -185)
  line L7 (500, -185) -> (0, -185)
  line L8 (0, -185) -> (0, -15)
  line L9 (0, -15) -> (20, -15)
  line L10 (20, -15) -> (20, -165)
  line L11 (20, -165) -> (480, -165)
  line L12 (480, -165) -> (480, -15)
  dimension "d127" = 35
  dimension "d128" = 20
  dimension "d129" = 150
  dimension "d130" = 460
  constraint coincident L1.end L2.start
  constraint perpendicular L1 L4
  constraint horizontal L5
  constraint vertical L6
  constraint horizontal L7
  constraint vertical L8
  constraint coincident L0.start L3.end
  constraint perpendicular L2 L9
  constraint perpendicular L9 L10
  constraint perpendicular L10 L11
  constraint coincident L5 L12.end
  constraint perpendicular L5 L12
  measures "d127" distance of L1.end L4.end
  measures "d128" distance of L4.end L9.end
  measures "d129" distance of L9.end L10.end
  measures "d130" distance of L10.end L11.end
move_face "DécalerLesFaces1" offset 140 1 faces at (166.6667, -35, 826.6667) on bodies 14
extrude "Extrusion33" cut sketch "Esquisse31" against normal blind 490 contours L5 L10 L11 L12 bodies 14